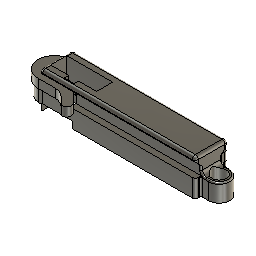
Pi Connector Cover 4 v4 (Autodesk Fusion 360 design; units mm, degrees)
Autodesk Fusion 360 part; units mm, degrees
sketch "Sketch1" plane through (0, 0, 0) normal (0, 0, 1) x (1, 0, 0)
  line L0 (25.4, -2.54) -> (-25.4, -2.54) construction
  line L1 (-25.4, -2.54) -> (-25.4, 2.54) construction
  line L2 (-25.4, 2.54) -> (25.4, 2.54) construction
  line L3 (25.4, 2.54) -> (25.4, -2.54) construction
  line L4 (25.4, -2.54) -> (-25.4, 2.54) construction
  line L5 (-25.4, -2.54) -> (25.4, 2.54) construction
  line L6 (29, 0) -> (-29, 0) construction
  line L7 (-25.79, -3.24) -> (-15.24, -3.24) construction
  line L8 (-15.24, -3.24) -> (-15.24, -16.24) construction
  line L9 (-15.24, -16.24) -> (-25.79, -16.24) construction
  line L10 (-25.79, -16.24) -> (-25.79, -3.24) construction
  line L11 (-23.805, -1.595) -> (-24.455, -1.595) construction
  line L12 (-24.455, -1.595) -> (-24.455, -0.945) construction
  line L13 (-24.455, -0.945) -> (-23.805, -0.945) construction
  line L14 (-23.805, -0.945) -> (-23.805, -1.595) construction
  line L15 (-23.805, -1.595) -> (-24.455, -0.945) construction
  line L16 (-24.455, -1.595) -> (-23.805, -0.945) construction
  line L17 (-21.915, -0.945) -> (-21.265, -0.945) construction
  line L18 (-21.915, -1.595) -> (-21.915, -0.945) construction
  line L19 (-21.265, -1.595) -> (-21.915, -1.595) construction
  line L20 (-21.265, -0.945) -> (-21.265, -1.595) construction
  line L21 (-19.375, -0.945) -> (-18.725, -0.945) construction
  line L22 (-19.375, -1.595) -> (-19.375, -0.945) construction
  line L23 (-18.725, -1.595) -> (-19.375, -1.595) construction
  line L24 (-18.725, -0.945) -> (-18.725, -1.595) construction
  line L25 (-16.835, -0.945) -> (-16.185, -0.945) construction
  line L26 (-16.835, -1.595) -> (-16.835, -0.945) construction
  line L27 (-16.185, -1.595) -> (-16.835, -1.595) construction
  line L28 (-16.185, -0.945) -> (-16.185, -1.595) construction
  line L29 (-14.295, -0.945) -> (-13.645, -0.945) construction
  line L30 (-14.295, -1.595) -> (-14.295, -0.945) construction
  line L31 (-13.645, -1.595) -> (-14.295, -1.595) construction
  line L32 (-13.645, -0.945) -> (-13.645, -1.595) construction
  line L33 (-11.755, -0.945) -> (-11.105, -0.945) construction
  line L34 (-11.755, -1.595) -> (-11.755, -0.945) construction
  line L35 (-11.105, -1.595) -> (-11.755, -1.595) construction
  line L36 (-11.105, -0.945) -> (-11.105, -1.595) construction
  line L37 (-9.215, -0.945) -> (-8.565, -0.945) construction
  line L38 (-9.215, -1.595) -> (-9.215, -0.945) construction
  line L39 (-8.565, -1.595) -> (-9.215, -1.595) construction
  line L40 (-8.565, -0.945) -> (-8.565, -1.595) construction
  line L41 (-6.675, -0.945) -> (-6.025, -0.945) construction
  line L42 (-6.675, -1.595) -> (-6.675, -0.945) construction
  line L43 (-6.025, -1.595) -> (-6.675, -1.595) construction
  line L44 (-6.025, -0.945) -> (-6.025, -1.595) construction
  line L45 (-4.135, -0.945) -> (-3.485, -0.945) construction
  line L46 (-4.135, -1.595) -> (-4.135, -0.945) construction
  line L47 (-3.485, -1.595) -> (-4.135, -1.595) construction
  line L48 (-3.485, -0.945) -> (-3.485, -1.595) construction
  line L49 (-1.595, -0.945) -> (-0.945, -0.945) construction
  line L50 (-1.595, -1.595) -> (-1.595, -0.945) construction
  line L51 (-0.945, -1.595) -> (-1.595, -1.595) construction
  line L52 (-0.945, -0.945) -> (-0.945, -1.595) construction
  line L53 (0.945, -0.945) -> (1.595, -0.945) construction
  line L54 (0.945, -1.595) -> (0.945, -0.945) construction
  line L55 (1.595, -1.595) -> (0.945, -1.595) construction
  line L56 (1.595, -0.945) -> (1.595, -1.595) construction
  line L57 (3.485, -0.945) -> (4.135, -0.945) construction
  line L58 (3.485, -1.595) -> (3.485, -0.945) construction
  line L59 (4.135, -1.595) -> (3.485, -1.595) construction
  line L60 (4.135, -0.945) -> (4.135, -1.595) construction
  line L61 (6.025, -0.945) -> (6.675, -0.945) construction
  line L62 (6.025, -1.595) -> (6.025, -0.945) construction
  line L63 (6.675, -1.595) -> (6.025, -1.595) construction
  line L64 (6.675, -0.945) -> (6.675, -1.595) construction
  line L65 (8.565, -0.945) -> (9.215, -0.945) construction
  line L66 (8.565, -1.595) -> (8.565, -0.945) construction
  line L67 (9.215, -1.595) -> (8.565, -1.595) construction
  line L68 (9.215, -0.945) -> (9.215, -1.595) construction
  line L69 (11.105, -0.945) -> (11.755, -0.945) construction
  line L70 (11.105, -1.595) -> (11.105, -0.945) construction
  line L71 (11.755, -1.595) -> (11.105, -1.595) construction
  line L72 (11.755, -0.945) -> (11.755, -1.595) construction
  line L73 (13.645, -0.945) -> (14.295, -0.945) construction
  line L74 (13.645, -1.595) -> (13.645, -0.945) construction
  line L75 (14.295, -1.595) -> (13.645, -1.595) construction
  line L76 (14.295, -0.945) -> (14.295, -1.595) construction
  line L77 (16.185, -0.945) -> (16.835, -0.945) construction
  line L78 (16.185, -1.595) -> (16.185, -0.945) construction
  line L79 (16.835, -1.595) -> (16.185, -1.595) construction
  line L80 (16.835, -0.945) -> (16.835, -1.595) construction
  line L81 (18.725, -0.945) -> (19.375, -0.945) construction
  line L82 (18.725, -1.595) -> (18.725, -0.945) construction
  line L83 (19.375, -1.595) -> (18.725, -1.595) construction
  line L84 (19.375, -0.945) -> (19.375, -1.595) construction
  line L85 (21.265, -0.945) -> (21.915, -0.945) construction
  line L86 (21.265, -1.595) -> (21.265, -0.945) construction
  line L87 (21.915, -1.595) -> (21.265, -1.595) construction
  line L88 (21.915, -0.945) -> (21.915, -1.595) construction
  line L89 (23.805, -0.945) -> (24.455, -0.945) construction
  line L90 (23.805, -1.595) -> (23.805, -0.945) construction
  line L91 (24.455, -1.595) -> (23.805, -1.595) construction
  line L92 (24.455, -0.945) -> (24.455, -1.595) construction
  line L93 (-24.455, 1.595) -> (-23.805, 1.595) construction
  line L94 (-24.455, 0.945) -> (-24.455, 1.595) construction
  line L95 (-23.805, 0.945) -> (-24.455, 0.945) construction
  line L96 (-23.805, 1.595) -> (-23.805, 0.945) construction
  line L97 (-21.915, 1.595) -> (-21.265, 1.595) construction
  line L98 (-21.915, 0.945) -> (-21.915, 1.595) construction
  line L99 (-21.265, 0.945) -> (-21.915, 0.945) construction
  line L100 (-21.265, 1.595) -> (-21.265, 0.945) construction
  line L101 (-19.375, 1.595) -> (-18.725, 1.595) construction
  line L102 (-19.375, 0.945) -> (-19.375, 1.595) construction
  line L103 (-18.725, 0.945) -> (-19.375, 0.945) construction
  line L104 (-18.725, 1.595) -> (-18.725, 0.945) construction
  line L105 (-16.835, 1.595) -> (-16.185, 1.595) construction
  line L106 (-16.835, 0.945) -> (-16.835, 1.595) construction
  line L107 (-16.185, 0.945) -> (-16.835, 0.945) construction
  line L108 (-16.185, 1.595) -> (-16.185, 0.945) construction
  line L109 (-14.295, 1.595) -> (-13.645, 1.595) construction
  line L110 (-14.295, 0.945) -> (-14.295, 1.595) construction
  line L111 (-13.645, 0.945) -> (-14.295, 0.945) construction
  line L112 (-13.645, 1.595) -> (-13.645, 0.945) construction
  line L113 (-11.755, 1.595) -> (-11.105, 1.595) construction
  line L114 (-11.755, 0.945) -> (-11.755, 1.595) construction
  line L115 (-11.105, 0.945) -> (-11.755, 0.945) construction
  line L116 (-11.105, 1.595) -> (-11.105, 0.945) construction
  line L117 (-9.215, 1.595) -> (-8.565, 1.595) construction
  line L118 (-9.215, 0.945) -> (-9.215, 1.595) construction
  line L119 (-8.565, 0.945) -> (-9.215, 0.945) construction
  line L120 (-8.565, 1.595) -> (-8.565, 0.945) construction
  line L121 (-6.675, 1.595) -> (-6.025, 1.595) construction
  line L122 (-6.675, 0.945) -> (-6.675, 1.595) construction
  line L123 (-6.025, 0.945) -> (-6.675, 0.945) construction
  line L124 (-6.025, 1.595) -> (-6.025, 0.945) construction
  line L125 (-4.135, 1.595) -> (-3.485, 1.595) construction
  line L126 (-4.135, 0.945) -> (-4.135, 1.595) construction
  line L127 (-3.485, 0.945) -> (-4.135, 0.945) construction
  line L128 (-3.485, 1.595) -> (-3.485, 0.945) construction
  line L129 (-1.595, 1.595) -> (-0.945, 1.595) construction
  line L130 (-1.595, 0.945) -> (-1.595, 1.595) construction
  line L131 (-0.945, 0.945) -> (-1.595, 0.945) construction
  line L132 (-0.945, 1.595) -> (-0.945, 0.945) construction
  line L133 (0.945, 1.595) -> (1.595, 1.595) construction
  line L134 (0.945, 0.945) -> (0.945, 1.595) construction
  line L135 (1.595, 0.945) -> (0.945, 0.945) construction
  line L136 (1.595, 1.595) -> (1.595, 0.945) construction
  line L137 (3.485, 1.595) -> (4.135, 1.595) construction
  line L138 (3.485, 0.945) -> (3.485, 1.595) construction
  line L139 (4.135, 0.945) -> (3.485, 0.945) construction
  line L140 (4.135, 1.595) -> (4.135, 0.945) construction
  line L141 (6.025, 1.595) -> (6.675, 1.595) construction
  line L142 (6.025, 0.945) -> (6.025, 1.595) construction
  line L143 (6.675, 0.945) -> (6.025, 0.945) construction
  line L144 (6.675, 1.595) -> (6.675, 0.945) construction
  line L145 (8.565, 1.595) -> (9.215, 1.595) construction
  line L146 (8.565, 0.945) -> (8.565, 1.595) construction
  line L147 (9.215, 0.945) -> (8.565, 0.945) construction
  line L148 (9.215, 1.595) -> (9.215, 0.945) construction
  line L149 (11.105, 1.595) -> (11.755, 1.595) construction
  line L150 (11.105, 0.945) -> (11.105, 1.595) construction
  line L151 (11.755, 0.945) -> (11.105, 0.945) construction
  line L152 (11.755, 1.595) -> (11.755, 0.945) construction
  line L153 (13.645, 1.595) -> (14.295, 1.595) construction
  line L154 (13.645, 0.945) -> (13.645, 1.595) construction
  line L155 (14.295, 0.945) -> (13.645, 0.945) construction
  line L156 (14.295, 1.595) -> (14.295, 0.945) construction
  line L157 (16.185, 1.595) -> (16.835, 1.595) construction
  line L158 (16.185, 0.945) -> (16.185, 1.595) construction
  line L159 (16.835, 0.945) -> (16.185, 0.945) construction
  line L160 (16.835, 1.595) -> (16.835, 0.945) construction
  line L161 (18.725, 1.595) -> (19.375, 1.595) construction
  line L162 (18.725, 0.945) -> (18.725, 1.595) construction
  line L163 (19.375, 0.945) -> (18.725, 0.945) construction
  line L164 (19.375, 1.595) -> (19.375, 0.945) construction
  line L165 (21.265, 1.595) -> (21.915, 1.595) construction
  line L166 (21.265, 0.945) -> (21.265, 1.595) construction
  line L167 (21.915, 0.945) -> (21.265, 0.945) construction
  line L168 (21.915, 1.595) -> (21.915, 0.945) construction
  line L169 (23.805, 1.595) -> (24.455, 1.595) construction
  line L170 (23.805, 0.945) -> (23.805, 1.595) construction
  line L171 (24.455, 0.945) -> (23.805, 0.945) construction
  line L172 (24.455, 1.595) -> (24.455, 0.945) construction
  point P0 (-24.13, -1.27)
  dimension "d8" = 50.8
  dimension "d9" = 5.08
  dimension "d10" = 58
  dimension "d11" = 10.55
  dimension "d12" = 13
  dimension "d13" = 0.7
  dimension "d14" = 0.39
  dimension "d25" = 0.65
  dimension "d26" = 0.65
  dimension "d28" = 1.27
  dimension "d29" = 1.27
  dimension "d32" = 2.54
  dimension "d33" = 2.54
  constraint perpendicular L0 L1
  constraint parallel L0 L2
  constraint parallel L1 L3
  constraint horizontal L0
  constraint coincident L4 origin
  constraint coincident L5 origin
  constraint perpendicular L1 L6
  constraint midpoint L6 origin
  constraint horizontal L7
  constraint vertical L8
  constraint horizontal L9
  constraint vertical L10
  constraint perpendicular L11 L12
  constraint parallel L11 L13
  constraint parallel L12 L14
  constraint horizontal L11
  constraint coincident L15 P0
  constraint coincident L16 P0
  measures "d8" distance of L1.end L2.end
  measures "d9" distance of L0.end L1.end
  measures "d10" distance of L6.start L6.end
  measures "d11" distance of L7.start L7.end
  measures "d12" distance of L7.start L9.end
  measures "d13" vertical distance of L0.end L7.start
  measures "d14" horizontal distance of L0.end L7.start
  measures "d25" distance of L12.end L13.end
  measures "d26" distance of L11.end L12.end
  measures "d28" distance of L1 P0
  measures "d29" distance of L6 P0
sketch "Sketch2" plane through (0, 0, 0) normal (0, 0, 1) x (1, 0, 0)
  line L0 (25.4, -2.54) -> (-25.4, -2.54)
  line L1 (25.4, 2.54) -> (25.4, -2.54)
  line L2 (-25.4, 2.54) -> (25.4, 2.54)
  line L3 (-25.4, -2.54) -> (-25.4, 2.54)
  line L4 (-26.4, 3.54) -> (26.4, 3.54)
  line L5 (26.4, 3.54) -> (26.4, -3.54)
  line L6 (26.4, -3.54) -> (-26.4, -3.54)
  line L7 (-26.4, -3.54) -> (-26.4, 3.54)
sketch "Sketch3" plane through (0, 0, 0) normal (0, 0, 1) x (1, 0, 0)
  line L0 (29, 0) -> (-29, 0)
  arc A0 (-24.8725, -1.27) -> (-23.3875, -1.27) centre (-24.13, -1.27) ccw
  line L1 (-24.13, -1.27) -> (-24.8725, -1.27) construction
  line L2 (-24.13, -1.27) -> (-23.3875, -1.27) construction
  arc A1 (-23.3875, 1.27) -> (-24.8725, 1.27) centre (-24.13, 1.27) ccw
  line L3 (-23.3875, 1.27) -> (-23.3875, -1.27)
  line L4 (-24.8725, 1.27) -> (-24.8725, -1.27)
  line L5 (-22.3325, 1.27) -> (-22.3325, -1.27)
  arc A2 (-20.8475, 1.27) -> (-22.3325, 1.27) centre (-21.59, 1.27) ccw
  line L6 (-20.8475, 1.27) -> (-20.8475, -1.27)
  arc A3 (-22.3325, -1.27) -> (-20.8475, -1.27) centre (-21.59, -1.27) ccw
  line L7 (-19.7925, 1.27) -> (-19.7925, -1.27)
  arc A4 (-18.3075, 1.27) -> (-19.7925, 1.27) centre (-19.05, 1.27) ccw
  line L8 (-18.3075, 1.27) -> (-18.3075, -1.27)
  arc A5 (-19.7925, -1.27) -> (-18.3075, -1.27) centre (-19.05, -1.27) ccw
  line L9 (-17.2525, 1.27) -> (-17.2525, -1.27)
  arc A6 (-15.7675, 1.27) -> (-17.2525, 1.27) centre (-16.51, 1.27) ccw
  line L10 (-15.7675, 1.27) -> (-15.7675, -1.27)
  arc A7 (-17.2525, -1.27) -> (-15.7675, -1.27) centre (-16.51, -1.27) ccw
  line L11 (-14.7125, 1.27) -> (-14.7125, -1.27)
  arc A8 (-13.2275, 1.27) -> (-14.7125, 1.27) centre (-13.97, 1.27) ccw
  line L12 (-13.2275, 1.27) -> (-13.2275, -1.27)
  arc A9 (-14.7125, -1.27) -> (-13.2275, -1.27) centre (-13.97, -1.27) ccw
  line L13 (-12.1725, 1.27) -> (-12.1725, -1.27)
  arc A10 (-10.6875, 1.27) -> (-12.1725, 1.27) centre (-11.43, 1.27) ccw
  line L14 (-10.6875, 1.27) -> (-10.6875, -1.27)
  arc A11 (-12.1725, -1.27) -> (-10.6875, -1.27) centre (-11.43, -1.27) ccw
  line L15 (-9.6325, 1.27) -> (-9.6325, -1.27)
  arc A12 (-8.1475, 1.27) -> (-9.6325, 1.27) centre (-8.89, 1.27) ccw
  line L16 (-8.1475, 1.27) -> (-8.1475, -1.27)
  arc A13 (-9.6325, -1.27) -> (-8.1475, -1.27) centre (-8.89, -1.27) ccw
  line L17 (-7.0925, 1.27) -> (-7.0925, -1.27)
  arc A14 (-5.6075, 1.27) -> (-7.0925, 1.27) centre (-6.35, 1.27) ccw
  line L18 (-5.6075, 1.27) -> (-5.6075, -1.27)
  arc A15 (-7.0925, -1.27) -> (-5.6075, -1.27) centre (-6.35, -1.27) ccw
  line L19 (-4.5525, 1.27) -> (-4.5525, -1.27)
  arc A16 (-3.0675, 1.27) -> (-4.5525, 1.27) centre (-3.81, 1.27) ccw
  line L20 (-3.0675, 1.27) -> (-3.0675, -1.27)
  arc A17 (-4.5525, -1.27) -> (-3.0675, -1.27) centre (-3.81, -1.27) ccw
  line L21 (-2.0125, 1.27) -> (-2.0125, -1.27)
  arc A18 (-0.5275, 1.27) -> (-2.0125, 1.27) centre (-1.27, 1.27) ccw
  line L22 (-0.5275, 1.27) -> (-0.5275, -1.27)
  arc A19 (-2.0125, -1.27) -> (-0.5275, -1.27) centre (-1.27, -1.27) ccw
  line L23 (0.5275, 1.27) -> (0.5275, -1.27)
  arc A20 (2.0125, 1.27) -> (0.5275, 1.27) centre (1.27, 1.27) ccw
  line L24 (2.0125, 1.27) -> (2.0125, -1.27)
  arc A21 (0.5275, -1.27) -> (2.0125, -1.27) centre (1.27, -1.27) ccw
  line L25 (3.0675, 1.27) -> (3.0675, -1.27)
  arc A22 (4.5525, 1.27) -> (3.0675, 1.27) centre (3.81, 1.27) ccw
  line L26 (4.5525, 1.27) -> (4.5525, -1.27)
  arc A23 (3.0675, -1.27) -> (4.5525, -1.27) centre (3.81, -1.27) ccw
  line L27 (5.6075, 1.27) -> (5.6075, -1.27)
  arc A24 (7.0925, 1.27) -> (5.6075, 1.27) centre (6.35, 1.27) ccw
  line L28 (7.0925, 1.27) -> (7.0925, -1.27)
  arc A25 (5.6075, -1.27) -> (7.0925, -1.27) centre (6.35, -1.27) ccw
  line L29 (8.1475, 1.27) -> (8.1475, -1.27)
  arc A26 (9.6325, 1.27) -> (8.1475, 1.27) centre (8.89, 1.27) ccw
  line L30 (9.6325, 1.27) -> (9.6325, -1.27)
  arc A27 (8.1475, -1.27) -> (9.6325, -1.27) centre (8.89, -1.27) ccw
  line L31 (10.6875, 1.27) -> (10.6875, -1.27)
  arc A28 (12.1725, 1.27) -> (10.6875, 1.27) centre (11.43, 1.27) ccw
  line L32 (12.1725, 1.27) -> (12.1725, -1.27)
  arc A29 (10.6875, -1.27) -> (12.1725, -1.27) centre (11.43, -1.27) ccw
  line L33 (13.2275, 1.27) -> (13.2275, -1.27)
  arc A30 (14.7125, 1.27) -> (13.2275, 1.27) centre (13.97, 1.27) ccw
  line L34 (14.7125, 1.27) -> (14.7125, -1.27)
  arc A31 (13.2275, -1.27) -> (14.7125, -1.27) centre (13.97, -1.27) ccw
  line L35 (15.7675, 1.27) -> (15.7675, -1.27)
  arc A32 (17.2525, 1.27) -> (15.7675, 1.27) centre (16.51, 1.27) ccw
  line L36 (17.2525, 1.27) -> (17.2525, -1.27)
  arc A33 (15.7675, -1.27) -> (17.2525, -1.27) centre (16.51, -1.27) ccw
  line L37 (18.3075, 1.27) -> (18.3075, -1.27)
  arc A34 (19.7925, 1.27) -> (18.3075, 1.27) centre (19.05, 1.27) ccw
  line L38 (19.7925, 1.27) -> (19.7925, -1.27)
  arc A35 (18.3075, -1.27) -> (19.7925, -1.27) centre (19.05, -1.27) ccw
  line L39 (20.8475, 1.27) -> (20.8475, -1.27)
  arc A36 (22.3325, 1.27) -> (20.8475, 1.27) centre (21.59, 1.27) ccw
  line L40 (22.3325, 1.27) -> (22.3325, -1.27)
  arc A37 (20.8475, -1.27) -> (22.3325, -1.27) centre (21.59, -1.27) ccw
  line L41 (23.3875, 1.27) -> (23.3875, -1.27)
  arc A38 (24.8725, 1.27) -> (23.3875, 1.27) centre (24.13, 1.27) ccw
  line L42 (24.8725, 1.27) -> (24.8725, -1.27)
  arc A39 (23.3875, -1.27) -> (24.8725, -1.27) centre (24.13, -1.27) ccw
  point P0 (-24.13, -1.27)
  dimension "d34" = 180
  dimension "d35" = 0.7425
  dimension "d38" = 2.54
  dimension "d39" = 0
  constraint coincident P0 A0.centre
  constraint symmetric L0 A0.start A1.end
  constraint symmetric L0 A0.end A1.start
  constraint symmetric L0 A0 A1
  constraint tangent A0 L3
  measures "d34" angle of L1 L2
  measures "d35" distance of P0 A0.end
extrude "Extrude1" add sketch "Sketch2" along normal blind 5 contours L0 L1 L2 L3 makes body 1
draft "Draft1" angle -45 neutral plane through (0, 0, 0) pull (0, 0, -1) 1 faces at (8.4667, -2.54, 1.6667) on bodies 1
draft "Draft2" angle -45 neutral plane through (0, 0, 0) pull (0, 0, -1) 1 faces at (-8.4667, 2.54, 1.6667) on bodies 1
extrude "Extrude3" add sketch "Sketch3" along normal blind 7 bodies 1
extrude "Extrude2" add sketch "Sketch2" along normal blind 10 separate body contours L0 L1 L2 L3 | L4 L5 L6 L7 makes body 2
combine "Combine1" operation cut target body 2 tool bodies 1
ref_plane "WorkPlane1" through (0, 0, -2.29) normal (0, 0, -1) x (-1, 0, 0)
sketch "Sketch4" plane through (0, 0, -2.29) normal (0, 0, -1) x (1, 0, 0)
  line L0 (29, 0) -> (-29, 0)
  line L1 (-25.4, 2.54) -> (-25.4, -2.54)
  line L2 (25.4, 2.54) -> (-25.4, 2.54)
  line L3 (-25.4, -2.54) -> (25.4, -2.54)
  line L4 (25.4, -2.54) -> (25.4, 2.54)
  line L5 (25.4, 3.54) -> (-25.4, 3.54)
  line L6 (-25.4, -3.54) -> (25.4, -3.54)
  arc A0 (-29, 3.54) -> (-29, -3.54) centre (-29, 0) ccw
  line L7 (-25.4, 3.54) -> (-29, 3.54)
  line L8 (-25.4, -3.54) -> (-29, -3.54)
  arc A1 (29, -3.54) -> (29, 3.54) centre (29, 0) ccw
  line L9 (29, 3.54) -> (25.4, 3.54)
  line L10 (25.4, -3.54) -> (29, -3.54)
  dimension "d43" = 1
  dimension "d44" = 1
  constraint coincident L0.end A0.centre
  constraint collinear L5 L7
  constraint collinear L6 L8
  constraint tangent A0 L7
  constraint tangent A0 L8
  constraint coincident L0.start A1.centre
  constraint tangent A1 L9
  constraint collinear L5 L9
  constraint tangent A1 L10
  constraint coincident A1.start L10.end
  constraint collinear L6 L10
extrude "Extrude4" add sketch "Sketch4" against normal blind 6.05 bodies 2
sketch "Sketch6" plane through (0, 0, 3.76) normal (0, 0, 1) x (-1, 0, 0)
  line L0 (26.4, -3.54) -> (29, -3.54)
  arc A0 (29, -3.54) -> (29, 3.54) centre (29, 0) ccw
  line L1 (29, 3.54) -> (26.4, 3.54)
  line L2 (26.4, 3.54) -> (26.4, -3.54)
  point P0 (29, 0)
  point P1 (-29, 0)
hole "Hole1" at (29, 0, 3.76) at (-29, 0, 3.76) direction (0, 0, -1) diameter 2.8 end through all counterbore diameter 4.9 counterbore depth 5.05 bodies 2
sketch "Sketch15" plane through (0, 0, 0) normal (0, 0, 1) x (1, 0, 0)
  line L0 (26.4, -3.54) -> (-26.4, -3.54) construction
  line L1 (-26.4, -3.54) -> (-26.4, 3.54) construction
  line L2 (26.4, 3.54) -> (26.4, -3.54) construction
  line L3 (-26.4, 3.54) -> (26.4, 3.54) construction
  line L4 (-26.4, 3.54) -> (26.4, 3.54)
  line L5 (26.4, 3.54) -> (26.4, 5.54)
  line L6 (26.4, 5.54) -> (-26.4, 5.54)
  line L7 (-26.4, 5.54) -> (-26.4, 3.54)
  line L8 (-26.4, -3.54) -> (26.4, -3.54)
  line L9 (26.4, -3.54) -> (26.4, -5.54)
  line L10 (26.4, -5.54) -> (-26.4, -5.54)
  line L11 (-26.4, -5.54) -> (-26.4, -3.54)
  dimension "d111" = 2
  dimension "d112" = 2
  constraint perpendicular L4 L5
  constraint parallel L4 L6
  constraint parallel L5 L7
  constraint coincident L2.start L3.end
  constraint perpendicular L2 L4
  constraint coincident L1.end L3.start
  constraint perpendicular L8 L9
  constraint parallel L8 L10
  constraint parallel L9 L11
  constraint coincident L0.start L2.end
  constraint perpendicular L2 L8
  constraint coincident L0.end L1.start
  measures "d111" distance of L1.end L6.end
  measures "d112" distance of L0.end L10.end
extrude "Extrude14" add sketch "Sketch15" along normal up to surface (10 mm away) and the other way up to surface (2.29 mm away) bodies 2
sketch "Sketch5" plane through (0, 0, 10) normal (0, 0, 1) x (-1, 0, 0)
  line L0 (-26.4, 5.54) -> (-26.4, -5.54)
  line L1 (26.4, -5.54) -> (26.4, 5.54)
  line L2 (25.4, -2.54) -> (-25.4, -2.54) construction
  line L3 (25.4, 2.54) -> (25.4, -2.54) construction
  line L4 (-25.4, 2.54) -> (25.4, 2.54) construction
  line L5 (17.78, -2.54) -> (17.78, 2.54) construction
  line L6 (25.6, 2.74) -> (25.6, -2.74)
  line L7 (25.6, -2.74) -> (9.96, -2.74)
  line L8 (9.96, -2.74) -> (9.96, 2.74)
  line L9 (9.96, 2.74) -> (25.6, -2.74) construction
  line L10 (25.6, 2.74) -> (9.96, -2.74) construction
  line L11 (16.13, 2.74) -> (16.13, 4.24)
  line L12 (16.13, 4.24) -> (19.43, 4.24)
  line L13 (19.43, 4.24) -> (19.43, 2.74)
  line L14 (9.96, 2.74) -> (16.13, 2.74)
  line L15 (19.43, 2.74) -> (25.6, 2.74)
  line L16 (-26.4, -5.54) -> (26.4, -5.54)
  line L17 (26.4, 5.54) -> (-26.4, 5.54)
  point P0 (17.78, 0)
  point P1 (17.78, 3.464)
  point P2 (17.78, 4.24)
  dimension "d47" = 7.62
  dimension "d48" = 5.48
  dimension "d49" = 15.64
  dimension "d50" = 3.3
  dimension "d85" = 1.5
  constraint coincident L2 L5.start
  constraint coincident L4 L5.end
  constraint perpendicular L4 L5
  constraint perpendicular L6 L14
  constraint parallel L7 L14
  constraint parallel L6 L8
  constraint horizontal L14
  constraint coincident L9 P0
  constraint coincident L10 P0
  constraint midpoint L5 P0
  constraint parallel L11 L13
  constraint coincident L5 P1
  constraint coincident L13.end L14
  constraint collinear L14 L15
  constraint perpendicular L13 L15
  constraint perpendicular L11 L12
  constraint midpoint L12 P2
  constraint coincident L5 P2
  measures "d47" distance of L2.start L5.start
  measures "d48" distance of L6.start L6.end
  measures "d49" distance of L6.end L7.end
  measures "d50" distance of L11.end L12.end
  measures "d85" distance of L12.end L13.end
extrude "Extrude5" cut sketch "Sketch5" against normal blind 10 contours L6 L7 L8 L11 L12 L13 L14 L15 bodies 2
sketch "Sketch16" plane through (-26.4, 0, 0) normal (-1, 0, 0) x (0, -1, 0)
  line L0 (-3.54, 3.76) -> (3.54, 3.76)
  line L1 (3.54, 3.76) -> (3.54, -2.29)
  line L2 (3.54, -2.29) -> (5.54, -2.29)
  line L3 (5.54, -2.29) -> (5.54, 10)
  line L4 (5.54, 10) -> (-5.54, 10)
  line L5 (-5.54, 10) -> (-5.54, -2.29)
  line L6 (-5.54, -2.29) -> (-3.54, -2.29)
  line L7 (-3.54, -2.29) -> (-3.54, 3.76)
  line L8 (-5.54, 10) -> (-5.54, -2.29) construction
  line L9 (-5.54, 10) -> (5.54, 10) construction
  line L10 (5.54, 10) -> (5.54, -2.29) construction
  line L11 (5.54, 8.76) -> (3.54, 6.76)
  line L12 (3.54, 6.76) -> (3.54, 3.76)
  line L13 (3.54, 3.76) -> (5.54, 3.76)
  line L14 (5.54, 3.76) -> (5.54, 8.76)
  line L15 (16.24, 0) -> (3.24, 0)
  line L16 (-5.54, 8.76) -> (-3.54, 6.76)
  line L17 (-3.54, 6.76) -> (-3.54, 3.76)
  line L18 (-3.54, 3.76) -> (-5.54, 3.76)
  line L19 (-5.54, 3.76) -> (-5.54, 8.76)
  point P0 (-2.54, 0)
  dimension "d120" = 3.76
  dimension "d123" = 3.76
  dimension "d131" = 3
  dimension "d132" = 2
  dimension "d133" = 135
  dimension "d134" = 135
  dimension "d135" = 3
  dimension "d136" = 2
  constraint vertical L12
  constraint horizontal L13
  constraint vertical L14
  constraint coincident L3 L11.start
  constraint vertical L17
  constraint horizontal L18
  constraint vertical L19
  constraint coincident L8 L16.start
  measures "d120" distance of L13.end L15
  measures "d123" vertical distance of L18.end P0
  measures "d131" distance of L11.end L0.end
  measures "d132" distance of L0.end L13.end
  measures "d133" angle of L11 L12
  measures "d134" angle of L16 L17
  measures "d135" distance of L16.end L0.start
  measures "d136" distance of L0.start L18.end
extrude "Extrude15" cut sketch "Sketch16" against normal through all contours L5 L16 L17 L18 L19 bodies 2
extrude "Extrude16" cut sketch "Sketch16" against normal up to surface (52.8 mm away) contours L3 L11 L12 L13 L14 bodies 2
sketch "Sketch14" plane through (0, 0, -2.29) normal (0, 0, -1) x (1, 0, 0)
  arc A0 (-29, 3.54) -> (-29, -3.54) centre (-29, 0) ccw
  line L0 (-29, -3.54) -> (-26.4, -3.54)
  arc A1 (29, -3.54) -> (29, 3.54) centre (29, 0) ccw
  line L1 (29, 3.54) -> (26.4, 3.54)
  line L2 (25.4, 2.54) -> (25.4, -2.54)
  line L3 (25.4, -2.54) -> (-25.4, -2.54)
  line L4 (-25.4, -2.54) -> (-25.4, 2.54)
  line L5 (-25.4, 2.54) -> (25.4, 2.54)
  circle A2 centre (-29, 0) radius 1.4
  circle A3 centre (29, 0) radius 1.4
  line L6 (-15.24, 3.24) -> (-15.24, 16.24)
  line L7 (-15.24, 16.24) -> (-25.79, 16.24)
  line L8 (-25.79, 16.24) -> (-25.79, 3.24)
  line L9 (25.4, 2.54) -> (-25.4, 2.54)
  line L10 (-15.24, 3.24) -> (-15.24, 2.54)
  line L11 (-25.79, 3.24) -> (-25.79, 2.54)
  line L12 (-25.79, 2.54) -> (-25.4, 2.54)
  line L13 (-26.4, -3.54) -> (-26.4, -5.54)
  line L14 (-26.4, -5.54) -> (26.4, -5.54)
  line L15 (26.4, -5.54) -> (26.4, -3.54)
  line L16 (26.4, -3.54) -> (29, -3.54)
  line L17 (26.4, 3.54) -> (26.4, 5.54)
  line L18 (26.4, 5.54) -> (-26.4, 5.54)
  line L19 (-26.4, 5.54) -> (-26.4, 3.54)
  line L20 (-26.4, 3.54) -> (-29, 3.54)
  constraint coincident L6.start L10.start
  constraint coincident L9 L10.end
  constraint coincident L8.end L11.start
  constraint perpendicular L9 L11
  constraint coincident L4.end L5.start
  constraint perpendicular L4 L12
  constraint collinear L6 L10
extrude "Extrude13" cut sketch "Sketch14" against normal up to surface (2.29 mm away) contours L5 L6 L8 L9 L10 L11 L12 L18 bodies 2
fillet "Fillet6" radius 1.5 1 edges at (26.4, 0, 3.76) on bodies 2
fillet "Fillet7" radius 1 12 edges at (-26.4, 0, 10) (0, 5.54, 10) (26.4, 0, 10) (0, -5.54, 10) (-26.4, 5.54, 9.38) (-26.4, 5.54, 0.735) (-26.4, -5.54, 9.38) (-26.4, -5.54, 0.735) (26.4, 5.54, 9.38) (26.4, 5.54, 0.735) (26.4, -5.54, 9.38) (26.4, -5.54, 0.735) on bodies 2
fillet "Fillet9" radius 0.5 2 edges at (-26.4, -3.54, 5.26) (-26.4, 3.54, 5.26) on bodies 2
fillet "Fillet10" radius 0.5 10 edges at (26.4, -3.54, 6.01) (26.8393, -3.54, 4.1993) (28.45, -3.54, 3.76) (32.54, 0, 3.76) (28.45, 3.54, 3.76) (26.8393, 3.54, 4.1993) (26.4, 3.54, 6.01) (-27.7, 3.54, 3.76) (-32.54, 0, 3.76) (-27.7, -3.54, 3.76) on bodies 2
fillet "Fillet11" radius 0.5 6 edges at (26.4, -3.54, 0.735) (26.4, 3.54, 0.735) (-26.4, 3.3936, 3.6136) (-26.4, 3.54, 0.485) (-26.4, -3.54, 0.485) (-26.4, -3.3936, 3.6136) on bodies 2
sketch "Sketch17" plane through (0, 0, 3.76) normal (0, 0, 1) x (-1, 0, 0)
  circle A0 centre (29, 0) radius 2.45
  line L0 (26.4, 3.906) -> (26.4, 4.54)
  line L1 (25.4, 5.54) -> (-25.4, 5.54)
  line L2 (-26.4, 4.54) -> (-26.4, 4.0204)
  spline S0 degree 3 poles (-26.8133, 3.5177) (-26.7512, 3.5289) (-26.6919, 3.5522) (-26.5827, 3.6211) (-26.5343, 3.667) (-26.4653, 3.7637) (-26.4414, 3.8111) (-26.4085, 3.9126) (-26.4, 3.9663) (-26.4, 4.0204) knots 0 0 0 0 0.018944 0.018944 0.038743 0.038743 0.054556 0.054556 0.070751 0.070751 0.070751 0.070751
  spline S1 degree 3 poles (-26.5771, 3.54) (-26.6555, 3.54) (-26.7344, 3.532) (-26.8133, 3.5177) knots 0.312946 0.312946 0.312946 0.312946 0.336448 0.336448 0.336448 0.336448
  line L3 (-26.5771, 3.54) -> (16.13, 3.54)
  line L4 (16.13, 3.54) -> (16.13, 4.24)
  line L5 (16.13, 4.24) -> (19.43, 4.24)
  line L6 (19.43, 4.24) -> (19.43, 3.54)
  line L7 (19.43, 3.54) -> (25.9, 3.54)
  arc A1 (26.4, 3.04) -> (25.9, 3.54) centre (25.9, 3.04) ccw
  line L8 (26.4, 3.04) -> (26.4, -3.04)
  arc A2 (25.9, -3.54) -> (26.4, -3.04) centre (25.9, -3.04) ccw
  line L9 (25.9, -3.54) -> (-26.5771, -3.54)
  spline S2 degree 3 poles (-26.8133, -3.5177) (-26.7344, -3.532) (-26.6555, -3.54) (-26.5771, -3.54) knots 0.113056 0.113056 0.113056 0.113056 0.136559 0.136559 0.136559 0.136559
  spline S3 degree 3 poles (-26.4, -4.0204) (-26.4, -3.9543) (-26.4128, -3.8887) (-26.4622, -3.766) (-26.4985, -3.7099) (-26.5806, -3.6249) (-26.6223, -3.5932) (-26.7136, -3.5441) (-26.7625, -3.5269) (-26.8133, -3.5177) knots 0 0 0 0 0.019832 0.019832 0.039683 0.039683 0.055294 0.055294 0.070789 0.070789 0.070789 0.070789
  line L10 (-25.4, -5.54) -> (25.4, -5.54)
  line L11 (26.4, -4.54) -> (26.4, -3.906)
  spline S4 degree 3 poles (26.9, -3.04) (26.7615, -3.1785) (26.598, -3.3476) (26.4448, -3.6324) (26.4, -3.7786) (26.4, -3.906) knots 0 0 0 0 0.058781 0.058781 0.097013 0.097013 0.097013 0.097013
  line L12 (26.9, -3.04) -> (29, -3.04)
  arc A3 (29, -3.04) -> (29, 3.04) centre (29, 0) ccw
  line L13 (29, 3.04) -> (26.9, 3.04)
  spline S5 degree 3 poles (26.4, 3.906) (26.4, 3.7786) (26.4448, 3.6324) (26.598, 3.3476) (26.7615, 3.1785) (26.9, 3.04) knots 0.252766 0.252766 0.252766 0.252766 0.290998 0.290998 0.349779 0.349779 0.349779 0.349779
  line L14 (-26.4, -5.54) -> (26.4, -5.54)
  line L15 (26.4, -3.54) -> (-26.4, -3.54)
  line L16 (-26.4, -3.54) -> (-26.4, -5.54)
  arc A4 (29, -3.54) -> (29, 3.54) centre (29, 0) ccw construction
  line L17 (26.4, 3.54) -> (-26.4, 3.54) construction
  line L18 (-26.4, 5.54) -> (26.4, 5.54) construction
  arc A5 (27, -5.54) -> (27, 5.54) centre (27, 0) ccw
  line L19 (26.4, -5.54) -> (27, -5.54)
  line L20 (26.4, 5.54) -> (27, 5.54)
  line L21 (26.4, -3.54) -> (26.4, 3.54)
  line L22 (19.43, 4.24) -> (19.43, 2.74) construction
  line L23 (26.4, 3.54) -> (19.43, 3.54)
  line L24 (19.43, 3.54) -> (19.43, 2.74)
  line L25 (17.93, 2.74) -> (13.6907, 6.9793)
  arc A6 (15.3126, 9.431) -> (13.6907, 6.9793) centre (14.7513, 8.04) ccw
  line L26 (15.3126, 9.431) -> (19.2036, 5.54)
  line L27 (17.93, 2.74) -> (19.43, 2.74)
  line L28 (19.2036, 5.54) -> (26.4, 5.54)
  arc A7 (26.4, 4.54) -> (25.4, 5.54) centre (25.4, 4.54) ccw
  arc A8 (-25.4, 5.54) -> (-26.4, 4.54) centre (-25.4, 4.54) ccw
  line L29 (-26.4, -4.0204) -> (-26.4, -4.54)
  arc A9 (-26.4, -4.54) -> (-25.4, -5.54) centre (-25.4, -4.54) ccw
  arc A10 (25.4, -5.54) -> (26.4, -4.54) centre (25.4, -4.54) ccw
  dimension "d143" = 1.5
  dimension "d144" = 135
  dimension "d145" = 1.5
  dimension "d146" = 2.5
  constraint coincident L14.end L19.start
  constraint coincident L18.end L20.start
  constraint collinear L14 L19
  constraint collinear L18 L20
  constraint tangent A5 L19
  constraint tangent A5 L20
  constraint tangent A4 A5
  constraint coincident L15.start L21.start
  constraint coincident L17.start L21.end
  constraint coincident L6.end L7.start
  constraint coincident L22.end L24.end
  constraint tangent L25 A6
  constraint coincident L1 L26.end
  constraint perpendicular L22 L27
  constraint parallel L18 L28
  constraint parallel L25 L26
  measures "d143" distance of L22.end L25.start
  measures "d144" angle of L25 L27
  measures "d145" radius of A6
  measures "d146" distance of L1 A6.centre
extrude "Extrude17" add sketch "Sketch17" along normal blind 3 separate body contours A0 | L0 L1 L5 L6 L7 L8 L9 L10 L11 S4 L12 A3 L13 S5 L14 L15 L16 L21 L23 L25 L28 A7 L29 A9 A10 | L0 L11 S4 L12 A3 L13 S5 L14 A5 L19 L20 L28 A7 A10 | L1 L25 A6 L26 | L5 L6 L24 L25 L27 makes body 3
fillet "Fillet12" radius 5 1 edges at (-19.2036, -5.54, 5.26) on bodies 3
fillet "Fillet13" radius 0.5 2 edges at (-26.4, 3.54, 5.26) (-26.4, -3.54, 5.26) on bodies 3
equation "M25_loose = 2.8 mm"
equation "M25_head_diam = 4.9 mm"
equation "body_clearance = 0.2 mm"
equation "pin_width = 0.65 mm"
equation "pin_clearance = 0.2 mm"
equation "pin_pitch = 0.1 in"
equation "row_count = 6"
equation "d8 = 20 * pin_pitch"
equation "d9 = 2 * pin_pitch"
equation "wall_thickness = 1 mm"
equation "d16 = -wall_thickness"
equation "d23 = body_height"
equation "d25 = pin_width"
equation "d26 = pin_width"
equation "d28 = pin_pitch / 2"
equation "d29 = pin_pitch / 2"
equation "d32 = pin_pitch"
equation "d33 = pin_pitch"
equation "d35 = ( pin_width + 2 * pin_clearance ) * sqrt(1 / 2)"
equation "d38 = pin_pitch"
equation "d42 = header_height"
equation "d43 = wall_thickness"
equation "d44 = wall_thickness"
equation "d45 = -shoulder_height"
equation "d47 = row_count * pin_pitch / 2"
equation "d48 = 2 * pin_pitch + 2 * body_clearance"
equation "d49 = row_count * pin_pitch + 2 * body_clearance"
equation "d50 = 2.5 mm + 4 * body_clearance"
equation "d52 = -body_height"
equation "d55 = M25_loose"
equation "d57 = shoulder_height - wall_thickness"
equation "d58 = M25_head_diam"
equation "shoulder_height = header_height + PV_key_height"
equation "PV_key_height = 3.76 mm"
equation "body_height = 10 mm"
equation "d120 = PV_key_height"
equation "d123 = d120"
equation "header_height = 2.29 mm"
named bodies: "Pi Connector Cover", "Pi Connector Clip"
